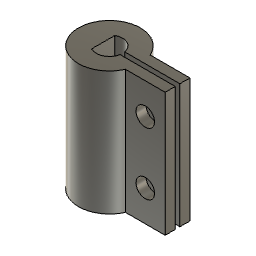
shaft_extender (Autodesk Fusion 360 design; units mm, degrees)
Autodesk Fusion 360 part; units mm, degrees
sketch "Sketch1" plane through (0, 0, 0) normal (0, 0, 1) x (1, 0, 0)
  circle A0 centre (0, 0) radius 5
  line L0 (11, 2.0022) -> (-1, 2.0022)
  line L1 (-1, 2.0022) -> (-1, -2.0022)
  line L2 (-1, -2.0022) -> (11, -2.0022)
  line L3 (11, -2.0022) -> (11, 2.0022)
  line L4 (11, 2.0022) -> (-1, -2.0022) construction
  line L5 (-1, 2.0022) -> (11, -2.0022) construction
  line L6 (11, 0) -> (5, 0) construction
  circle A1 centre (0, 0) radius 2.125
  line L7 (-1, 1.875) -> (-1, -1.875)
  circle A2 centre (0, 0) radius 2.6
  line L8 (13.9695, 0.375) -> (-3.9695, 0.375)
  line L9 (-3.9695, 0.375) -> (-3.9695, -0.375)
  line L10 (-3.9695, -0.375) -> (13.9695, -0.375)
  line L11 (13.9695, -0.375) -> (13.9695, 0.375)
  line L12 (13.9695, 0.375) -> (-3.9695, -0.375) construction
  line L13 (-3.9695, 0.375) -> (13.9695, -0.375) construction
  line L14 (5, 0) -> (0, 0) construction
  point P0 (5, 0)
  point P1 (5, 0)
  dimension "d1" = 10
  dimension "d2" = 6
  dimension "d3" = 4.25
  dimension "d4" = 1
  dimension "d5" = 5.2
  dimension "d6" = 0.75
  constraint coincident A0.centre A1.centre
  constraint horizontal L0
  constraint perpendicular L0 L1
  constraint parallel L0 L2
  constraint parallel L1 L3
  constraint coincident L4 P1
  constraint coincident L5 P1
  constraint coincident A0 P1
  constraint midpoint L3 L6.start
  constraint coincident P1 P0
  constraint coincident A1 L7.start
  constraint coincident A1 L7.end
  constraint vertical L7
  constraint concentric A1 A2
  constraint horizontal L8
  constraint perpendicular L8 L9
  constraint parallel L8 L10
  constraint parallel L9 L11
  constraint coincident L12 P1
  constraint coincident L13 P1
  constraint horizontal L14
  measures "d1" diameter of A0
  measures "d2" distance of L6.start P1
  measures "d3" diameter of A1
  measures "d4" distance of A0.centre L7
  measures "d5" diameter of A2
  measures "d6" distance of L8 L10
extrude "Extrude1" add sketch "Sketch1" along normal blind 10 contours A0 L0 A2 L8 | A0 L0 L3 L8 | A0 L2 L3 L10 | A0 L2 A2 L10 | A0 L0 L2 A2 L8 L9 L10 | L0 A1 A2 L8 | L2 A1 A2 L10 | L0 L1 A1 A2 L8 | L1 L2 A1 A2 L10 | A1 A2 L8 L10 | A2 L8 L9 L10 | L1 A1 L7 L8 | L1 A1 L7 L8 L10 | L1 A1 L7 L10 | L0 L1 A1 | L1 L2 A1 picked at (-2.2619, -0.2919) picked at (-1.3738, -0.0419)
extrude "Extrude2" add sketch "Sketch1" against normal blind 10 contours A0 L0 A2 L8 | A0 L0 L3 L8 | A0 L2 L3 L10 | A0 L2 A2 L10 | A0 L0 L2 A2 L8 L9 L10 | A2 L8 L9 L10
sketch "Sketch2" plane through (0, -2.0022, 0) normal (0, -1, 0) x (1, 0, 0)
  line L0 (11, -10) -> (11, 10)
  line L1 (11, 10) -> (4.5816, 10)
  line L2 (4.5816, 10) -> (4.5816, -10)
  line L3 (4.5816, -10) -> (11, -10)
  line L4 (11, -10) -> (4.5816, 10) construction
  line L5 (7.7908, 0) -> (11, 0) construction
  line L6 (11, 0) -> (4.5816, 10) construction
  line L7 (11, 0) -> (4.5816, -10) construction
  circle A0 centre (7.7908, -5) radius 1.5
  circle A1 centre (7.7908, 5) radius 1.5
  dimension "d11" = 3
  constraint coincident L0.start L3.end
  constraint coincident L1.end L2.start
  constraint midpoint L4 L5.start
  constraint midpoint L0 L5.end
  constraint coincident L2.end L3.start
  constraint midpoint L7 A0.centre
  constraint midpoint L6 A1.centre
  constraint equal A0 A1
  measures "d11" diameter of A0
extrude "Extrude3" cut sketch "Sketch2" against normal blind 5 contours A0 | A1
sketch "Sketch3" plane through (11, 0, 0) normal (1, 0, 0) x (0, 1, 0)
  line L0 (2.0022, -10) -> (2.0022, 10)
  line L1 (-0.375, 10) -> (-2.0022, 10)
  line L2 (-2.0022, 10) -> (-2.0022, -10)
  line L3 (-2.0022, -10) -> (-0.375, -10)
  line L4 (-0.375, -10) -> (-2.0022, 10) construction
  line L5 (-0.2455, -10) -> (0.2455, -10) construction
  line L6 (0.2455, -10) -> (0.2455, 10)
  line L7 (0.2455, 10) -> (-0.2455, 10) construction
  line L8 (-0.2455, 10) -> (-0.2455, -10)
  line L9 (-0.2455, -10) -> (0.2455, 10) construction
  line L10 (0.2455, -10) -> (-0.2455, 10) construction
  line L11 (-0.375, -10) -> (-0.375, 10)
  line L12 (0.375, 10) -> (0.375, -10)
  line L13 (2.0022, 10) -> (0.375, 10)
  line L14 (0.375, -10) -> (2.0022, -10)
  constraint coincident L3.end L4.start
  constraint coincident L1.end L2.start
  constraint horizontal L5
  constraint perpendicular L5 L6
  constraint parallel L5 L7
  constraint parallel L6 L8
  constraint coincident L9 origin
  constraint coincident L10 origin
  constraint coincident L3 L5.start
